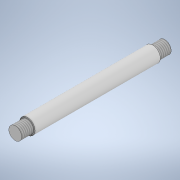
# Autodesk Inventor part: Eje roscado base soporte tubo
Saved by Autodesk Inventor 2021 (Build 250183000, 183)
## iProperties
Created: 2021-05-29
Part Number: Eje roscado base soporte tubo
Material: Generic
Document SubType Name: Modeling
Designer: Nelson
Density: 1 g/cm^3
Appearance: Default
Author: Nelson
Autodesk Inventor part; units mm, degrees
ref_plane "YZ Plane" through (0, 0, 0) normal (1, 0, 0) x (0, 1, 0)
ref_plane "XZ Plane" through (0, 0, 0) normal (0, 1, 0) x (-1, 0, 0)
ref_plane "XY Plane" through (0, 0, 0) normal (0, 0, 1) x (1, 0, 0)
sketch "Sketch2" plane through (0, 0, 0) normal (1, 0, 0) x (0, 1, 0)
  line L0 (0, 0) -> (7.9375, 0)
  line L1 (7.9375, 0) -> (7.9375, -15)
  line L2 (7.9375, -15) -> (9.525, -15)
  line L3 (9.525, -15) -> (9.525, -170)
  line L4 (9.525, -170) -> (7.9375, -170)
  line L5 (7.9375, -170) -> (7.9375, -185)
  line L6 (7.9375, -185) -> (0, -185)
  line L7 (0, -185) -> (0, 0)
  dimension "d7" = 7.9375
  dimension "d8" = 15
  dimension "d9" = 1.5875
  dimension "d10" = 15
  dimension "d11" = 1.5875
  dimension "d12" = 7.9375
  dimension "d13" = 155
  constraints: 16 end point, 5 perpendicular, 2 horizontal, 1 vertical
  measures "d7" distance of L0.start L0.end
  measures "d8" distance of L0.end L1.end
  measures "d9" distance of L1.end L2.end
  measures "d10" distance of L4.end L5.end
  measures "d11" distance of L3.end L4.end
  measures "d12" distance of L5.end L6.end
  measures "d13" distance of L2.end L3.end
revolve "Revolution1" add sketch "Sketch2" angle 360 about axis through (0, 0, -185) along (0, 0, 1)
thread "Thread4" size "5/8-11 UNC" class "2A" standard "ANSI Unified Screw Threads" full length
thread "Thread5" size "5/8-11 UNC" class "2A" standard "ANSI Unified Screw Threads" full length
equation "\"d10\" = d8"
equation "\"d11\" = d9"
body "Solid2"
